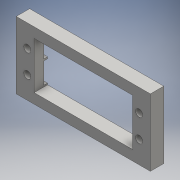
# Autodesk Inventor part: servoHolderTest1
Saved by Autodesk Inventor 2016 (Build 200138000, 138)
## iProperties
Created: 2016-04-16
Part Number: servoHolderTest1
Material: Generic
Document SubType Name: Modeling
Designer: hesaon
Density: 1 g/cm^3
Appearance: Default
Author: hesaon
Autodesk Inventor part; units mm, degrees
ref_plane "YZ Plane" through (0, 0, 0) normal (1, 0, 0) x (0, 1, 0)
ref_plane "XZ Plane" through (0, 0, 0) normal (0, 1, 0) x (-1, 0, 0)
ref_plane "XY Plane" through (0, 0, 0) normal (0, 0, 1) x (1, 0, 0)
sketch "Sketch1" plane through (0, 0, 0) normal (0, 1, 0) x (-1, 0, 0)
  line L0 (0, 0) -> (60, 0)
  line L1 (60, 0) -> (60, -30)
  line L2 (60, -30) -> (0, -30)
  line L3 (0, -30) -> (0, 0)
  line L4 (52, -4.5) -> (8, -4.5)
  line L5 (8, -4.5) -> (8, -25.5)
  line L6 (8, -25.5) -> (52, -25.5)
  line L7 (52, -25.5) -> (52, -4.5)
  circle A0 centre (55, -9.9) radius 1.6
  circle A1 centre (55, -20.1) radius 1.6
  circle A2 centre (5, -9.9) radius 1.6
  circle A3 centre (5, -20.1) radius 1.6
  dimension "d0" = 60
  dimension "d1" = 30
  dimension "d2" = 44
  dimension "d3" = 21
  dimension "d4" = 8
  dimension "d5" = 4.5
  dimension "d6" = 3.2
  dimension "d7" = 3.2
  dimension "d8" = 5.4
  dimension "d9" = 3
  dimension "d10" = 3
  dimension "d11" = 5.4
  dimension "d12" = 3.2
  dimension "d13" = 3.2
  dimension "d15" = 5.4
  dimension "d16" = 5.4
  dimension "d47" = 3
  dimension "d48" = 3
  constraints: 16 end point, 4 centre point, 4 parallel, 2 horizontal, 2 perpendicular
  measures "d0" distance of L1.end L2.end
  measures "d1" distance of L0.end L1.end
  measures "d2" distance of L4.end L4.start
  measures "d3" distance of L5.end L4.end
  measures "d4" distance from line of L3 L4.end
  measures "d5" distance from line of L0 L4.end
  measures "d6" diameter of A0
  measures "d7" diameter of A1
  measures "d8" distance from line of A0.centre L4
  measures "d9" distance from line of L7 A0.centre
  measures "d10" distance from line of L7 A1.centre
  measures "d11" distance from line of L6 A1.centre
  measures "d12" diameter of A2
  measures "d13" diameter of A3
  measures "d15" distance from line of L6 A3.centre
  measures "d16" distance from line of L4 A2.centre
  measures "d47" distance from line of L5 A2.centre
  measures "d48" distance from line of L5 A3.centre
extrude "Extrusion1" add sketch "Sketch1" along normal blind 6
sketch "Sketch2" plane through (0, 6, 0) normal (0, 1, 0) x (1, 0, 0)
  line L0 (-8.2, 24.8) -> (-1.8, 24.8)
  line L1 (-1.8, 24.8) -> (-1.8, 15.4)
  line L2 (-1.8, 15.4) -> (-8.2, 15.4)
  line L3 (-8.2, 15.4) -> (-8.2, 24.8)
  line L4 (-8.2, 5.2) -> (-1.8, 5.2)
  line L5 (-1.8, 5.2) -> (-1.8, 14.6)
  line L6 (-1.8, 14.6) -> (-8.2, 14.6)
  line L7 (-8.2, 14.6) -> (-8.2, 5.2)
  line L8 (0, 0) -> (0, 30) projected
  line L9 (-60, 0) -> (0, 0) projected
  line L10 (-58.2, 5.2) -> (-51.8, 5.2)
  line L11 (-51.8, 5.2) -> (-51.8, 14.6)
  line L12 (-51.8, 14.6) -> (-58.2, 14.6)
  line L13 (-58.2, 14.6) -> (-58.2, 5.2)
  line L14 (-58.2, 15.4) -> (-51.8, 15.4)
  line L15 (-51.8, 15.4) -> (-51.8, 24.8)
  line L16 (-51.8, 24.8) -> (-58.2, 24.8)
  line L17 (-58.2, 24.8) -> (-58.2, 15.4)
  line L18 (-60, 0) -> (-60, 30) projected
  circle A0 centre (-55, 20.1) radius 1.6 projected
  circle A1 centre (-55, 9.9) radius 1.6 projected
  circle A2 centre (-5, 20.1) radius 1.6 projected
  circle A3 centre (-5, 9.9) radius 1.6 projected
  line L19 (-52, 4.5) -> (-52, 25.5) projected
  line L20 (-52, 25.5) -> (-8, 25.5) projected
  line L21 (-8, 25.5) -> (-8, 4.5) projected
  line L22 (-8, 4.5) -> (-52, 4.5) projected
  circle A4 centre (-5, 20.1) radius 1.6 projected
  circle A5 centre (-5, 9.9) radius 1.6 projected
  circle A6 centre (-55, 20.1) radius 1.6 projected
  circle A7 centre (-55, 9.9) radius 1.6 projected
  line L23 (-60, 0) -> (0, 0) projected
  line L24 (0, 0) -> (0, 30) projected
  line L25 (0, 30) -> (-60, 30) projected
  line L26 (-60, 30) -> (-60, 0) projected
  dimension "d32" = 6.4
  dimension "d37" = 6.4
  dimension "d38" = 9.4
  dimension "d49" = 9.4
  dimension "d50" = 9.4
  dimension "d51" = 9.4
  dimension "d52" = 6.4
  dimension "d53" = 6.4
  dimension "d54" = 4.7
  dimension "d55" = 4.7
  dimension "d56" = 3.2
  dimension "d57" = 3.2
  dimension "d58" = 4.7
  dimension "d60" = 3.2
  dimension "d61" = 3.2
  dimension "d62" = 4.7
  constraints: 32 end point, 8 parallel, 4 horizontal, 4 perpendicular
  measures "d32" distance of L4.end L4.start
  measures "d37" distance of L12.end L11.end
  measures "d38" distance of L11.end L10.end
  measures "d49" distance of L15.end L14.end
  measures "d50" distance of L1.end L0.end
  measures "d51" distance of L5.end L4.end
  measures "d52" distance of L0.end L0.start
  measures "d53" distance of L15.end L16.end
  measures "d54" distance from line of L16 A0.centre
  measures "d55" distance from line of L10 A1.centre
  measures "d56" distance from line of L11 A1.centre
  measures "d57" distance from line of L15 A0.centre
  measures "d58" distance from line of L4 A3.centre
  measures "d60" distance from line of L3 A4.centre
  measures "d61" distance from line of L7 A3.centre
  measures "d62" vertical distance of L0.end A2.centre
extrude "Extrusion2" cut sketch "Sketch2" against normal blind 1.6 contours L0 L21 L2 L3 | L0 L1 L2 L21 | L21 L4 L7 L6 | L6 L5 L4 L21 | L19 L14 L17 L16 | L16 L15 L14 L19 | L19 L10 L13 L12 | L12 L11 L10 L19 | A0 | A1 | A2 | A3
body "Solid1"
